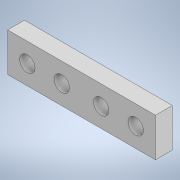
# Autodesk Inventor part: switch_mount
Saved by Autodesk Inventor 2022.2 (Build 262287000, 287)
## iProperties
Created: 2022-01-24
Part Number: switch_mount
Material: Generic
Document SubType Name: Modeling
Designer: hugof
Density: 1 g/cm^3
Appearance: Default
Author: hugof
Autodesk Inventor part; units mm, degrees
ref_plane "YZ Plane" through (0, 0, 0) normal (1, 0, 0) x (0, 1, 0)
ref_plane "XZ Plane" through (0, 0, 0) normal (0, 1, 0) x (-1, 0, 0)
ref_plane "XY Plane" through (0, 0, 0) normal (0, 0, 1) x (1, 0, 0)
sketch "Sketch1" plane through (0, 0, 0) normal (0, 0, 1) x (1, 0, 0)
  line L0 (0, 0) -> (-29.8, 0)
  line L1 (0, 15.6035) -> (0, 0)
  circle A0 centre (-7.95, 7.8017) radius 5.95
  circle A1 centre (-21.85, 7.8017) radius 5.95
  line L2 (-29.8, 15.6035) -> (-29.8, 0)
  line L3 (-29.8, 15.6035) -> (0, 15.6035)
  line L4 (-29.8, 0) -> (-60, 0)
  line L5 (-21.85, 7.8017) -> (-21.85, 15.6035)
  line L6 (-21.85, 7.8017) -> (-21.85, 0)
  line L7 (-7.95, 7.8017) -> (-7.95, 0)
  line L8 (-7.95, 7.8017) -> (-7.95, 15.6035)
  line L9 (-59.6, 0) -> (-29.8, 0)
  line L10 (-59.6, 15.6035) -> (-59.6, 0)
  circle A2 centre (-51.65, 7.8017) radius 5.95
  circle A3 centre (-37.75, 7.8017) radius 5.95
  line L11 (-29.8, 15.6035) -> (-59.6, 15.6035)
  line L12 (-37.75, 7.8017) -> (-37.75, 15.6035)
  line L13 (-37.75, 7.8017) -> (-37.75, 0)
  line L14 (-51.65, 7.8017) -> (-51.65, 0)
  line L15 (-51.65, 7.8017) -> (-51.65, 15.6035)
  point P0 (0, 7.8017)
  point P1 (-59.6, 7.8017)
  dimension "d0" = 11.9
  dimension "d1" = 11.9
  dimension "d7" = 7.95
  dimension "d8" = 13.9
  dimension "d9" = 7.95
  constraints: 32 end point, 12 point on line, 9 symmetric about line, 4 centre point, 4 perpendicular, 3 parallel, 2 collinear, 2 horizontal, 1 midpoint, 2 other
  measures "d0" diameter of A0
  measures "d1" diameter of A1
  measures "d7" distance from line of L2 L5.start
  measures "d8" distance of L7.start L5.start
  measures "d9" distance from line of L1 L7.start
extrude "Extrusion1" add sketch "Sketch1" along normal blind 0.8 contours L0 L7 A0 L8 L3 L1 | L0 L6 A1 L5 L3 L8 A0 L7 | L0 L2 L3 L5 A1 L6 | L4 L13 A3 L12 L11 L2 | L4 L14 A2 L15 L11 L12 A3 L13 | L4 L10 L11 L15 A2 L14
sketch "Sketch2" plane through (0, 0, 0.8) normal (0, 0, 1) x (1, 0, 0)
  line L0 (-59.6, 15.6035) -> (-59.6, 0) projected
  line L1 (-59.6, 0) -> (0, 0) projected
  line L2 (-59.6, 15.6035) -> (0, 15.6035)
  line L3 (0, 15.6035) -> (0, 0)
  line L4 (0, 0) -> (-59.6, 0)
  line L5 (-59.6, 0) -> (-59.6, 15.6035)
  constraints: 8 end point, 2 parallel, 1 horizontal, 1 perpendicular
extrude "Extrusion2" add sketch "Sketch2" along normal blind 6
sketch "Sketch3" plane through (-7.95, 7.8017, 0.8) normal (0, 0, -1) x (-1, 0, 0)
  circle A0 centre (0, 0) radius 5.95 projected
  line L0 (0, 0) -> (-4.55, 0)
  line L1 (0, 0) -> (4.55, 0)
  line L2 (0, 0) -> (0, 4.55)
  line L3 (0, 0) -> (0, -4.55)
  line L4 (-4.55, 0) -> (-4.55, -1.8847)
  line L5 (0, 0) -> (2.5958, -2.5958)
  line L6 (0, 0) -> (3.671, 0) construction
  line L7 (3.2173, -3.2173) -> (-3.2173, 3.2173)
  line L8 (0, 0) -> (-3.2173, -3.2173)
  line L9 (0, 0) -> (3.2173, 3.2173)
  line L10 (-3.2173, -3.2173) -> (-1.8847, -4.55)
  line L11 (-3.2173, -3.2173) -> (-4.55, -1.8847)
  line L12 (3.2173, -3.2173) -> (1.8847, -4.55)
  line L13 (3.2173, -3.2173) -> (4.55, -1.8847)
  line L14 (4.55, 0) -> (4.55, -1.8847)
  line L15 (4.55, 0) -> (4.55, 1.8847)
  line L16 (3.2173, 3.2173) -> (4.55, 1.8847)
  line L17 (3.2173, 3.2173) -> (1.8847, 4.55)
  line L18 (0, 4.55) -> (1.8847, 4.55)
  line L19 (0, 4.55) -> (-1.8847, 4.55)
  line L20 (-3.2173, 3.2173) -> (-1.8847, 4.55)
  line L21 (-3.2173, 3.2173) -> (-4.55, 1.8847)
  line L22 (0, -4.55) -> (1.8847, -4.55)
  line L23 (0, -4.55) -> (-1.8847, -4.55)
  line L24 (-4.55, 0) -> (-4.55, 1.8847)
  line L25 (5.95, 0) -> (7.95, 0)
  circle A1 centre (13.9, 0) radius 5.95 projected
  line L26 (6.95, 0) -> (6.95, 2.7112)
  line L27 (-7.95, 7.8017) -> (51.65, 7.8017) projected
  circle A2 centre (13.9, 0) radius 5.95
  line L28 (13.9, 0) -> (18.45, 0)
  line L29 (13.9, 0) -> (9.35, 0)
  line L30 (13.9, 0) -> (13.9, 4.55)
  line L31 (13.9, 0) -> (13.9, -4.55)
  line L32 (18.45, 0) -> (18.45, -1.8847)
  line L33 (13.9, 0) -> (11.3042, -2.5958)
  line L34 (13.9, 0) -> (10.229, 0) construction
  line L35 (10.6827, -3.2173) -> (17.1173, 3.2173)
  line L36 (13.9, 0) -> (17.1173, -3.2173)
  line L37 (13.9, 0) -> (10.6827, 3.2173)
  line L38 (17.1173, -3.2173) -> (15.7847, -4.55)
  line L39 (17.1173, -3.2173) -> (18.45, -1.8847)
  line L40 (10.6827, -3.2173) -> (12.0153, -4.55)
  line L41 (10.6827, -3.2173) -> (9.35, -1.8847)
  line L42 (9.35, 0) -> (9.35, -1.8847)
  line L43 (9.35, 0) -> (9.35, 1.8847)
  line L44 (10.6827, 3.2173) -> (9.35, 1.8847)
  line L45 (10.6827, 3.2173) -> (12.0153, 4.55)
  line L46 (13.9, 4.55) -> (12.0153, 4.55)
  line L47 (13.9, 4.55) -> (15.7847, 4.55)
  line L48 (17.1173, 3.2173) -> (15.7847, 4.55)
  line L49 (17.1173, 3.2173) -> (18.45, 1.8847)
  line L50 (13.9, -4.55) -> (12.0153, -4.55)
  line L51 (13.9, -4.55) -> (15.7847, -4.55)
  line L52 (18.45, 0) -> (18.45, 1.8847)
  line L53 (21.85, 7.8017) -> (21.85, -7.8017)
  line L54 (51.65, -7.8017) -> (-7.95, -7.8017) projected
  circle A3 centre (43.7, 0) radius 5.95
  line L55 (43.7, 0) -> (48.25, 0)
  line L56 (43.7, 0) -> (39.15, 0)
  line L57 (43.7, 0) -> (43.7, 4.55)
  line L58 (43.7, 0) -> (43.7, -4.55)
  line L59 (48.25, 0) -> (48.25, -1.8847)
  line L60 (43.7, 0) -> (41.1042, -2.5958)
  line L61 (43.7, 0) -> (40.029, 0) construction
  line L62 (40.4827, -3.2173) -> (46.9173, 3.2173)
  line L63 (43.7, 0) -> (46.9173, -3.2173)
  line L64 (43.7, 0) -> (40.4827, 3.2173)
  line L65 (46.9173, -3.2173) -> (45.5847, -4.55)
  line L66 (46.9173, -3.2173) -> (48.25, -1.8847)
  line L67 (40.4827, -3.2173) -> (41.8153, -4.55)
  line L68 (40.4827, -3.2173) -> (39.15, -1.8847)
  line L69 (39.15, 0) -> (39.15, -1.8847)
  line L70 (39.15, 0) -> (39.15, 1.8847)
  line L71 (40.4827, 3.2173) -> (39.15, 1.8847)
  line L72 (40.4827, 3.2173) -> (41.8153, 4.55)
  line L73 (43.7, 4.55) -> (41.8153, 4.55)
  line L74 (43.7, 4.55) -> (45.5847, 4.55)
  line L75 (46.9173, 3.2173) -> (45.5847, 4.55)
  line L76 (46.9173, 3.2173) -> (48.25, 1.8847)
  line L77 (43.7, -4.55) -> (41.8153, -4.55)
  line L78 (43.7, -4.55) -> (45.5847, -4.55)
  line L79 (48.25, 0) -> (48.25, 1.8847)
  line L80 (37.75, 0) -> (35.75, 0)
  circle A4 centre (29.8, 0) radius 5.95
  line L81 (36.75, 0) -> (36.75, 2.7112)
  line L82 (25.25, 0) -> (25.25, 1.8847)
  line L83 (25.25, 0) -> (25.25, -1.8847)
  line L84 (29.8, 0) -> (25.25, 0)
  line L85 (29.8, 0) -> (29.8, 4.55)
  line L86 (29.8, 0) -> (29.8, -4.55)
  line L87 (29.8, -4.55) -> (27.9153, -4.55)
  line L88 (29.8, 4.55) -> (31.6847, 4.55)
  line L89 (29.8, 0) -> (33.0173, 3.2173)
  line L90 (29.8, 0) -> (32.3958, -2.5958)
  line L91 (29.8, -4.55) -> (31.6847, -4.55)
  line L92 (33.0173, 3.2173) -> (34.35, 1.8847)
  line L93 (34.35, 0) -> (34.35, -1.8847)
  line L94 (33.0173, -3.2173) -> (26.5827, 3.2173)
  line L95 (33.0173, -3.2173) -> (34.35, -1.8847)
  circle A5 centre (29.8, 0) radius 5.95
  line L96 (33.0173, -3.2173) -> (31.6847, -4.55)
  line L97 (29.8, 0) -> (34.35, 0)
  line L98 (34.35, 0) -> (34.35, 1.8847)
  line L99 (29.8, 0) -> (33.471, 0) construction
  line L100 (26.5827, 3.2173) -> (27.9153, 4.55)
  line L101 (33.0173, 3.2173) -> (31.6847, 4.55)
  line L102 (29.8, 4.55) -> (27.9153, 4.55)
  line L103 (26.5827, 3.2173) -> (25.25, 1.8847)
  line L104 (26.5827, -3.2173) -> (25.25, -1.8847)
  line L105 (26.5827, -3.2173) -> (27.9153, -4.55)
  line L106 (29.8, 0) -> (26.5827, -3.2173)
  dimension "d14" = 4.55
  dimension "d15" = 4.55
  dimension "d16" = 4.55
  dimension "d17" = 4.55
  dimension "d22" = 45
  constraints: 210 end point, 65 symmetric about line, 9 perpendicular, 9 vertical, 7 horizontal, 7 midpoint, 6 horizontal alignment, 4 coincident, 1 equal length, 10 other
  measures "d14" distance of L0.start L0.end
  measures "d15" distance of L0.start L1.end
  measures "d16" distance of L0.start L2.end
  measures "d17" distance of L0.start L3.end
  measures "d22" angle of L5 L6
sketch "Sketch4" plane through (-37.75, 7.8017, 0.8) normal (0, 0, -1) x (-1, 0, 0)
  line L0 (3.2173, -3.2173) -> (1.8847, -4.55) projected
  line L1 (3.2173, -3.2173) -> (4.55, -1.8847) projected
  line L2 (4.55, 0) -> (4.55, -1.8847) projected
  line L3 (4.55, 0) -> (4.55, 1.8847) projected
  line L4 (3.2173, 3.2173) -> (4.55, 1.8847) projected
  line L5 (3.2173, 3.2173) -> (1.8847, 4.55) projected
  line L6 (0, 4.55) -> (1.8847, 4.55) projected
  line L7 (0, 4.55) -> (-1.8847, 4.55) projected
  line L8 (-3.2173, 3.2173) -> (-1.8847, 4.55) projected
  line L9 (-3.2173, 3.2173) -> (-4.55, 1.8847) projected
  line L10 (-4.55, 0) -> (-4.55, 1.8847) projected
  line L11 (-4.55, 0) -> (-4.55, -1.8847) projected
  line L12 (-3.2173, -3.2173) -> (-4.55, -1.8847) projected
  line L13 (-3.2173, -3.2173) -> (-1.8847, -4.55) projected
  line L14 (0, -4.55) -> (-1.8847, -4.55) projected
  line L15 (0, -4.55) -> (1.8847, -4.55) projected
  line L16 (-4.55, 1.8847) -> (-4.55, -1.8847)
  line L17 (-1.8847, -4.55) -> (1.8847, -4.55)
  line L18 (4.55, -1.8847) -> (4.55, 1.8847)
  line L19 (1.8847, 4.55) -> (-1.8847, 4.55)
  line L20 (1.8847, -4.55) -> (4.55, -1.8847)
  line L21 (-1.8847, -4.55) -> (-4.55, -1.8847)
  line L22 (-4.55, 1.8847) -> (-1.8847, 4.55)
  line L23 (1.8847, 4.55) -> (4.55, 1.8847)
  circle A0 centre (0, 0) radius 5.95 projected
  circle A1 centre (0, 0) radius 5.95
  line L24 (10.6827, 3.2173) -> (12.0153, 4.55) projected
  line L25 (10.6827, 3.2173) -> (9.35, 1.8847) projected
  line L26 (9.35, 0) -> (9.35, 1.8847) projected
  line L27 (9.35, 0) -> (9.35, -1.8847) projected
  line L28 (10.6827, -3.2173) -> (9.35, -1.8847) projected
  line L29 (10.6827, -3.2173) -> (12.0153, -4.55) projected
  line L30 (13.9, -4.55) -> (12.0153, -4.55) projected
  line L31 (13.9, -4.55) -> (15.7847, -4.55) projected
  line L32 (17.1173, -3.2173) -> (15.7847, -4.55) projected
  line L33 (17.1173, -3.2173) -> (18.45, -1.8847) projected
  line L34 (18.45, 0) -> (18.45, -1.8847) projected
  line L35 (18.45, 0) -> (18.45, 1.8847) projected
  line L36 (17.1173, 3.2173) -> (18.45, 1.8847) projected
  line L37 (17.1173, 3.2173) -> (15.7847, 4.55) projected
  line L38 (13.9, 4.55) -> (15.7847, 4.55) projected
  line L39 (13.9, 4.55) -> (12.0153, 4.55) projected
  line L40 (9.35, 1.8847) -> (12.0153, 4.55)
  line L41 (12.0153, 4.55) -> (15.7847, 4.55)
  line L42 (15.7847, 4.55) -> (18.45, 1.8847)
  line L43 (18.45, 1.8847) -> (18.45, -1.8847)
  line L44 (18.45, -1.8847) -> (15.7847, -4.55)
  line L45 (9.35, -1.8847) -> (12.0153, -4.55)
  line L46 (-15.9, 4.55) -> (-17.7847, 4.55) projected
  line L47 (-15.9, 4.55) -> (-14.0153, 4.55) projected
  line L48 (-12.6827, 3.2173) -> (-14.0153, 4.55) projected
  line L49 (-12.6827, 3.2173) -> (-11.35, 1.8847) projected
  line L50 (-11.35, 0) -> (-11.35, 1.8847) projected
  line L51 (-11.35, 0) -> (-11.35, -1.8847) projected
  line L52 (-12.6827, -3.2173) -> (-11.35, -1.8847) projected
  line L53 (-12.6827, -3.2173) -> (-14.0153, -4.55) projected
  line L54 (-15.9, -4.55) -> (-14.0153, -4.55) projected
  line L55 (-15.9, -4.55) -> (-17.7847, -4.55) projected
  line L56 (-19.1173, -3.2173) -> (-17.7847, -4.55) projected
  line L57 (-19.1173, -3.2173) -> (-20.45, -1.8847) projected
  line L58 (-20.45, 0) -> (-20.45, -1.8847) projected
  line L59 (-20.45, 0) -> (-20.45, 1.8847) projected
  line L60 (-19.1173, 3.2173) -> (-20.45, 1.8847) projected
  line L61 (-19.1173, 3.2173) -> (-17.7847, 4.55) projected
  line L62 (-17.7847, 4.55) -> (-14.0153, 4.55)
  line L63 (-11.35, 1.8847) -> (-14.0153, 4.55)
  line L64 (-17.7847, 4.55) -> (-20.45, 1.8847)
  line L65 (-20.45, -1.8847) -> (-17.7847, -4.55)
  line L66 (-17.7847, -4.55) -> (-14.0153, -4.55)
  line L67 (-11.35, -1.8847) -> (-11.35, 1.8847)
  line L68 (-11.35, -1.8847) -> (-14.0153, -4.55)
  circle A2 centre (-15.9, 0) radius 5.95
  line L69 (-33.0173, 3.2173) -> (-34.35, 1.8847) projected
  line L70 (-33.0173, 3.2173) -> (-31.6847, 4.55) projected
  line L71 (-29.8, 4.55) -> (-31.6847, 4.55) projected
  line L72 (-29.8, 4.55) -> (-27.9153, 4.55) projected
  line L73 (-26.5827, 3.2173) -> (-27.9153, 4.55) projected
  line L74 (-26.5827, 3.2173) -> (-25.25, 1.8847) projected
  line L75 (-25.25, 0) -> (-25.25, 1.8847) projected
  line L76 (-25.25, 0) -> (-25.25, -1.8847) projected
  line L77 (-26.5827, -3.2173) -> (-25.25, -1.8847) projected
  line L78 (-26.5827, -3.2173) -> (-27.9153, -4.55) projected
  line L79 (-29.8, -4.55) -> (-27.9153, -4.55) projected
  line L80 (-29.8, -4.55) -> (-31.6847, -4.55) projected
  line L81 (-33.0173, -3.2173) -> (-31.6847, -4.55) projected
  line L82 (-33.0173, -3.2173) -> (-34.35, -1.8847) projected
  line L83 (-34.35, 0) -> (-34.35, -1.8847) projected
  line L84 (-34.35, 1.8847) -> (-31.6847, 4.55)
  line L85 (-27.9153, 4.55) -> (-25.25, 1.8847)
  line L86 (-25.25, -1.8847) -> (-27.9153, -4.55)
  line L87 (-31.6847, -4.55) -> (-27.9153, -4.55)
  line L88 (-34.35, -1.8847) -> (-31.6847, -4.55)
  line L89 (-34.35, -1.8847) -> (-34.35, 1.8847)
  circle A3 centre (-29.8, 0) radius 5.95
  circle A4 centre (13.9, 0) radius 5.95
  circle A5 centre (13.9, 0) radius 5.95
  line L90 (-31.6847, 4.55) -> (-27.9153, 4.55)
  line L91 (-25.25, 1.8847) -> (-25.25, -1.8847)
  line L92 (-20.45, -1.8847) -> (-20.45, 1.8847)
  line L93 (9.35, -1.8847) -> (9.35, 1.8847)
  line L94 (12.0153, -4.55) -> (15.7847, -4.55)
  point P0 (-37.75, -7.8017)
  constraints: 66 end point, 19 collinear, 6 perpendicular, 5 centre point, 3 point on line, 2 coincident, 2 parallel, 1 concentric, 1 horizontal
extrude "Extrusion3" cut sketch "Sketch4" against normal blind 1.5 contours L0 L15 L14 L13 L12 L11 L10 L9 L8 L7 L6 L5 L4 L3 L2 L1 | L24 L39 L38 L37 L36 L35 L34 L33 L32 L31 L30 L29 L28 L27 L26 L25 | L47 L48 L49 L50 L51 L52 L53 L54 L55 L56 L57 L58 L59 L60 L61 L46 | L70 L71 L72 L73 L74 L75 L76 L77 L78 L79 L80 L81 L82 L83 L89 L69
sketch "Sketch5" plane through (-37.75, 7.8017, 2.3) normal (0, 0, -1) x (-1, 0, 0)
  circle A0 centre (0, 0) radius 3.1
  circle A1 centre (0, 0) radius 3.1
  circle A2 centre (13.9, 0) radius 3.1
  circle A3 centre (-15.9, 0) radius 3.1
  circle A4 centre (-29.8, 0) radius 3.1
  line L0 (-25.25, 1.8847) -> (-25.25, -1.8847) projected
  line L1 (-34.35, -1.8847) -> (-34.35, 1.8847) projected
  line L2 (-25.25, -1.8847) -> (-27.9153, -4.55) projected
  circle A5 centre (-29.8, 0) radius 4.9249
  line L3 (-15.9, 0) -> (-20.45, 0)
  line L4 (-20.45, -1.8847) -> (-20.45, 1.8847) projected
  line L5 (-15.9, 0) -> (-11.35, 0)
  line L6 (-11.35, 1.8847) -> (-11.35, -1.8847) projected
  line L7 (0, 0) -> (-4.55, 0)
  line L8 (-4.55, -1.8847) -> (-4.55, 1.8847) projected
  line L9 (0, 0) -> (4.55, 0)
  line L10 (4.55, 1.8847) -> (4.55, -1.8847) projected
  line L11 (13.9, 0) -> (9.35, 0)
  line L12 (9.35, -1.8847) -> (9.35, 1.8847) projected
  line L13 (18.45, 1.8847) -> (18.45, -1.8847) projected
  line L14 (18.45, 0) -> (13.9, 0)
  point P0 (-37.75, -7.8017)
  dimension "d25" = 6.2
  dimension "d26" = 6.2
  dimension "d27" = 6.2
  dimension "d28" = 6.2
  dimension "d29" = 6.2
  constraints: 12 end point, 6 midpoint, 5 centre point, 3 collinear, 1 coincident, 1 perpendicular, 3 other
  measures "d25" diameter of A0
  measures "d26" diameter of A1
  measures "d27" diameter of A2
  measures "d28" diameter of A3
  measures "d29" diameter of A4
extrude "Extrusion4" cut sketch "Sketch5" against normal through all contours L9 L7 A0 | A0 L7 L9 | L14 L11 A2 | A2 L11 L14 | L5 L3 A3 | A3 L3 L5 | A4
body "Solid1"
